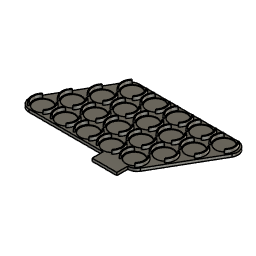
electrode_container_plate_rev_A_v1 (Autodesk Fusion 360 design; units mm, degrees)
Autodesk Fusion 360 part; units mm, degrees
note: some values were not read from the file. Chosen so that the rebuilt part matches the saved one: which bodies a step acts on. Set by a fixed rule: which sketch regions a step uses.
sketch "Sketch1" plane through (0, 0, 0) normal (0, 0, 1) x (1, 0, 0)
  circle A0 centre (0, 0) radius 8.55
  circle A1 centre (0, 0) radius 10
  line L0 (-7.0711, 7.0711) -> (7.0711, -7.0711)
  line L1 (-7.0711, -7.0711) -> (7.0711, 7.0711)
  line L2 (10, 0) -> (-10, 0) construction
  circle A2 centre (0, 0) radius 8
  dimension "d1" = 17.1
  dimension "d2" = 20
  dimension "d3" = 45
  dimension "d4" = 45
  dimension "d31" = 16
  constraint coincident A0.centre A1.centre
  constraint concentric A0 A1
  constraint coincident A1 L0.start
  constraint coincident A1 L0.end
  constraint coincident A1 L1.start
  constraint coincident A1 L1.end
  constraint midpoint A0.centre L1
  constraint midpoint A0.centre L0
  constraint coincident A1 L2.start
  constraint coincident A1 L2.end
  constraint horizontal L2
  measures "d1" diameter of A0
  measures "d2" diameter of A1
  measures "d3" angle of L1 L2
  measures "d4" angle of L0 L2
  measures "d31" diameter of A2
extrude "Extrude1" add sketch "Sketch1" along normal blind 3 draft -5 contours A0 A1 L0 L1 | A0 A1 L0 L1 picked at (9.4638, -0.8071) picked at (-7.307, -6.0626) makes body 1 at (9.2025, 3.6841, 1) makes body 2 at (-9.2025, 3.6841, 1)
pattern_linear "R-Pattern1" count 5 spacing 21 along (1, 0, 0) of bodies 2 1 makes body 3 at (30.2025, 3.6841, 1) makes body 4 at (51.2025, 3.6841, 1) makes body 5 at (72.2025, 3.6841, 1) makes body 6 at (93.2025, 3.6841, 1) makes body 7 at (11.7975, 3.6841, 1) makes body 8 at (32.7975, 3.6841, 1) makes body 9 at (53.7975, 3.6841, 1) makes body 10 at (74.7975, 3.6841, 1)
sketch "Sketch2" plane through (0, 0, 0) normal (0, 0, 1) x (1, 0, 0)
  line L0 (0, 0) -> (25.6285, 44.3898) construction
  line L1 (0, 0) -> (108.2634, 0) construction
  dimension "d11" = 60
  constraint coincident L0.start L1.start
  constraint horizontal L1
  measures "d11" angle of L0 L1
pattern_linear "R-Pattern2" count 4 spacing 20 along (0.5, 0.866025, 0) of bodies 6 1 3 5 10 2 7 9 8 4 makes body 11 at (19.2025, 21.0046, 1) makes body 12 at (29.2025, 38.3251, 1) makes body 13 at (39.2025, 55.6456, 1) makes body 14 at (0.7975, 21.0046, 1) makes body 15 at (10.7975, 38.3251, 1) makes body 16 at (20.7975, 55.6456, 1) makes body 17 at (40.2025, 21.0046, 1) makes body 18 at (50.2025, 38.3251, 1) makes body 19 at (60.2025, 55.6456, 1) makes body 20 at (61.2025, 21.0046, 1) makes body 21 at (71.2025, 38.3251, 1) makes body 22 at (81.2025, 55.6456, 1) makes body 23 at (82.2025, 21.0046, 1) makes body 24 at (92.2025, 38.3251, 1) makes body 25 at (102.2025, 55.6456, 1) makes body 26 at (103.2025, 21.0046, 1) makes body 27 at (113.2025, 38.3251, 1) makes body 28 at (123.2025, 55.6456, 1) makes body 29 at (21.7975, 21.0046, 1) makes body 30 at (31.7975, 38.3251, 1) makes body 31 at (41.7975, 55.6456, 1) makes body 32 at (42.7975, 21.0046, 1) makes body 33 at (52.7975, 38.3251, 1) makes body 34 at (62.7975, 55.6456, 1) makes body 35 at (63.7975, 21.0046, 1) makes body 36 at (73.7975, 38.3251, 1) makes body 37 at (83.7975, 55.6456, 1) makes body 38 at (84.7975, 21.0046, 1) makes body 39 at (94.7975, 38.3251, 1) makes body 40 at (104.7975, 55.6456, 1)
sketch "Sketch3" plane through (0, 0, 0) normal (0, 0, 1) x (1, 0, 0)
  line L0 (-18.2372, -9.0711) -> (22.2372, 61.0326)
  line L1 (22.2372, 61.0326) -> (132.2372, 61.0326)
  line L2 (132.2372, 61.0326) -> (91.7628, -9.0711)
  arc A0 (91.0686, -6.6974) -> (91.0686, 6.6974) centre (84, 0) ccw
  spline S0 degree 2 poles (91.0711, -7.0711) (91.0711, -6.883) (91.0686, -6.6974) knots 0.02979 0.02979 0.02979 0.332096 0.332096 0.332096
  arc A1 (91.0711, -7.0711) -> (91.0711, 7.0711) centre (84, 0) ccw
  spline S1 degree 2 poles (91.0711, 7.0711) (91.0711, 6.883) (91.0686, 6.6974) knots 0.02979 0.02979 0.02979 0.332096 0.332096 0.332096
  arc A2 (22.9314, 58.6589) -> (22.9314, 45.2641) centre (30, 51.9615) ccw
  spline S2 degree 2 poles (22.9289, 59.0326) (22.9289, 58.8445) (22.9314, 58.6589) knots 0.02979 0.02979 0.02979 0.332096 0.332096 0.332096
  arc A3 (22.9289, 59.0326) -> (22.9289, 44.8905) centre (30, 51.9615) ccw
  spline S3 degree 2 poles (22.9289, 44.8905) (22.9289, 45.0785) (22.9314, 45.2641) knots 0.02979 0.02979 0.02979 0.332096 0.332096 0.332096
  line L3 (94, 0) -> (97, 0) construction
  line L4 (20, 51.9615) -> (17, 51.9615) construction
  line L5 (-18.2372, -9.0711) -> (91.7628, -9.0711)
  point P0 (91.0711, -7.0711)
  point P1 (-7.0711, -7.0711)
  point P2 (22.9289, 59.0326)
  point P3 (20, 51.9615)
  point P4 (94, 0)
  dimension "d17" = 60
  dimension "d19" = 2
  dimension "d20" = 3
  dimension "d21" = 3
  dimension "d27" = 2
  dimension "d28" = 60
  constraint horizontal L1
  constraint midpoint A3 P3
  constraint midpoint A1 P4
  constraint coincident P4 L3.start
  constraint coincident L2 L3.end
  constraint horizontal L3
  constraint coincident P3 L4.start
  constraint coincident L0 L4.end
  constraint horizontal L4
  constraint horizontal L5
  constraint coincident L0.start L5.start
  measures "d17" angle of L1 L2
  measures "d19" distance of L1 P2
  measures "d20" distance of P3 L4.end
  measures "d21" distance of P4 L3.end
  measures "d27" distance of P1 L5
  measures "d28" angle of L0 L5
extrude "Extrude2" add sketch "Sketch3" against normal blind 2.5 contours L0 L1 L2 L5 | A0 S0 A1 S1 | A2 S2 A3 S3 bodies 1 2 3 4 5 6 7 8 9 10 11 12 13 14 15 16 17 18 19 20 21 22 23 24 25 26 27 28 29 30 31 32 33 34 35 36 37 38 39 40
sketch "Sketch4" plane through (0, 0, -2.5) normal (0, 0, -1) x (1, 0, 0)
  line L0 (91.7628, 9.0711) -> (-18.2372, 9.0711)
  line L1 (-18.2372, 9.0711) -> (22.2372, -61.0326)
  line L2 (22.2372, -61.0326) -> (132.2372, -61.0326)
  line L3 (132.2372, -61.0326) -> (91.7628, 9.0711)
  line L4 (96.9289, -41.7121) -> (97.9542, -40.6868)
  arc A0 (97.9542, -28.5953) -> (97.9542, -40.6868) centre (104, -34.641) ccw
  line L5 (97.9542, -28.5953) -> (96.9289, -27.5699)
  arc A1 (96.9289, -27.5699) -> (96.9289, -41.7121) centre (104, -34.641) ccw
  line L6 (85.9289, -59.0326) -> (86.9542, -58.0073)
  arc A2 (86.9542, -45.9158) -> (86.9542, -58.0073) centre (93, -51.9615) ccw
  line L7 (86.9542, -45.9158) -> (85.9289, -44.8905)
  arc A3 (85.9289, -44.8905) -> (85.9289, -59.0326) centre (93, -51.9615) ccw
  line L8 (65.9289, -24.3916) -> (66.9542, -23.3663)
  arc A4 (66.9542, -11.2747) -> (66.9542, -23.3663) centre (73, -17.3205) ccw
  line L9 (66.9542, -11.2747) -> (65.9289, -10.2494)
  arc A5 (65.9289, -10.2494) -> (65.9289, -24.3916) centre (73, -17.3205) ccw
  line L10 (54.9289, -41.7121) -> (55.9542, -40.6868)
  arc A6 (55.9542, -28.5953) -> (55.9542, -40.6868) centre (62, -34.641) ccw
  line L11 (55.9542, -28.5953) -> (54.9289, -27.5699)
  arc A7 (54.9289, -27.5699) -> (54.9289, -41.7121) centre (62, -34.641) ccw
  line L12 (43.9289, -59.0326) -> (44.9542, -58.0073)
  arc A8 (44.9542, -45.9158) -> (44.9542, -58.0073) centre (51, -51.9615) ccw
  line L13 (44.9542, -45.9158) -> (43.9289, -44.8905)
  arc A9 (43.9289, -44.8905) -> (43.9289, -59.0326) centre (51, -51.9615) ccw
  line L14 (23.9289, -24.3916) -> (24.9542, -23.3663)
  arc A10 (24.9542, -11.2747) -> (24.9542, -23.3663) centre (31, -17.3205) ccw
  line L15 (24.9542, -11.2747) -> (23.9289, -10.2494)
  arc A11 (23.9289, -10.2494) -> (23.9289, -24.3916) centre (31, -17.3205) ccw
  line L16 (111.0711, -27.5699) -> (110.0458, -28.5953)
  arc A12 (110.0458, -40.6868) -> (110.0458, -28.5953) centre (104, -34.641) ccw
  line L17 (110.0458, -40.6868) -> (111.0711, -41.7121)
  arc A13 (111.0711, -41.7121) -> (111.0711, -27.5699) centre (104, -34.641) ccw
  line L18 (100.0711, -44.8905) -> (99.0458, -45.9158)
  arc A14 (99.0458, -58.0073) -> (99.0458, -45.9158) centre (93, -51.9615) ccw
  line L19 (99.0458, -58.0073) -> (100.0711, -59.0326)
  arc A15 (100.0711, -59.0326) -> (100.0711, -44.8905) centre (93, -51.9615) ccw
  line L20 (80.0711, -10.2494) -> (79.0458, -11.2747)
  arc A16 (79.0458, -23.3663) -> (79.0458, -11.2747) centre (73, -17.3205) ccw
  line L21 (79.0458, -23.3663) -> (80.0711, -24.3916)
  arc A17 (80.0711, -24.3916) -> (80.0711, -10.2494) centre (73, -17.3205) ccw
  line L22 (69.0711, -27.5699) -> (68.0458, -28.5953)
  arc A18 (68.0458, -40.6868) -> (68.0458, -28.5953) centre (62, -34.641) ccw
  line L23 (68.0458, -40.6868) -> (69.0711, -41.7121)
  arc A19 (69.0711, -41.7121) -> (69.0711, -27.5699) centre (62, -34.641) ccw
  line L24 (58.0711, -44.8905) -> (57.0458, -45.9158)
  arc A20 (57.0458, -58.0073) -> (57.0458, -45.9158) centre (51, -51.9615) ccw
  line L25 (57.0458, -58.0073) -> (58.0711, -59.0326)
  arc A21 (58.0711, -59.0326) -> (58.0711, -44.8905) centre (51, -51.9615) ccw
  line L26 (38.0711, -10.2494) -> (37.0458, -11.2747)
  arc A22 (37.0458, -23.3663) -> (37.0458, -11.2747) centre (31, -17.3205) ccw
  line L27 (37.0458, -23.3663) -> (38.0711, -24.3916)
  arc A23 (38.0711, -24.3916) -> (38.0711, -10.2494) centre (31, -17.3205) ccw
  line L28 (12.9289, -41.7121) -> (13.9542, -40.6868)
  arc A24 (13.9542, -28.5953) -> (13.9542, -40.6868) centre (20, -34.641) ccw
  line L29 (13.9542, -28.5953) -> (12.9289, -27.5699)
  arc A25 (12.9289, -27.5699) -> (12.9289, -41.7121) centre (20, -34.641) ccw
  line L30 (37.0711, -44.8905) -> (36.0458, -45.9158)
  arc A26 (36.0458, -58.0073) -> (36.0458, -45.9158) centre (30, -51.9615) ccw
  line L31 (36.0458, -58.0073) -> (37.0711, -59.0326)
  arc A27 (37.0711, -59.0326) -> (37.0711, -44.8905) centre (30, -51.9615) ccw
  line L32 (17.0711, -10.2494) -> (16.0458, -11.2747)
  arc A28 (16.0458, -23.3663) -> (16.0458, -11.2747) centre (10, -17.3205) ccw
  line L33 (16.0458, -23.3663) -> (17.0711, -24.3916)
  arc A29 (17.0711, -24.3916) -> (17.0711, -10.2494) centre (10, -17.3205) ccw
  line L34 (55.9289, -7.0711) -> (56.9542, -6.0458)
  arc A30 (56.9542, 6.0458) -> (56.9542, -6.0458) centre (63, 0) ccw
  line L35 (56.9542, 6.0458) -> (55.9289, 7.0711)
  arc A31 (55.9289, 7.0711) -> (55.9289, -7.0711) centre (63, 0) ccw
  line L36 (13.9289, -7.0711) -> (14.9542, -6.0458)
  arc A32 (14.9542, 6.0458) -> (14.9542, -6.0458) centre (21, 0) ccw
  line L37 (14.9542, 6.0458) -> (13.9289, 7.0711)
  arc A33 (13.9289, 7.0711) -> (13.9289, -7.0711) centre (21, 0) ccw
  line L38 (70.0711, 7.0711) -> (69.0458, 6.0458)
  arc A34 (69.0458, -6.0458) -> (69.0458, 6.0458) centre (63, 0) ccw
  line L39 (69.0458, -6.0458) -> (70.0711, -7.0711)
  arc A35 (70.0711, -7.0711) -> (70.0711, 7.0711) centre (63, 0) ccw
  line L40 (28.0711, 7.0711) -> (27.0458, 6.0458)
  arc A36 (27.0458, -6.0458) -> (27.0458, 6.0458) centre (21, 0) ccw
  line L41 (27.0458, -6.0458) -> (28.0711, -7.0711)
  arc A37 (28.0711, -7.0711) -> (28.0711, 7.0711) centre (21, 0) ccw
  line L42 (7.0711, 7.0711) -> (6.0458, 6.0458)
  arc A38 (6.0458, -6.0458) -> (6.0458, 6.0458) centre (0, 0) ccw
  line L43 (6.0458, -6.0458) -> (7.0711, -7.0711)
  arc A39 (7.0711, -7.0711) -> (7.0711, 7.0711) centre (0, 0) ccw
  line L44 (-7.0711, -7.0711) -> (-6.0458, -6.0458)
  arc A40 (-6.0458, 6.0458) -> (-6.0458, -6.0458) centre (0, 0) ccw
  line L45 (-6.0458, 6.0458) -> (-7.0711, 7.0711)
  arc A41 (-7.0711, 7.0711) -> (-7.0711, -7.0711) centre (0, 0) ccw
  line L46 (49.0711, 7.0711) -> (48.0458, 6.0458)
  arc A42 (48.0458, -6.0458) -> (48.0458, 6.0458) centre (42, 0) ccw
  line L47 (48.0458, -6.0458) -> (49.0711, -7.0711)
  arc A43 (49.0711, -7.0711) -> (49.0711, 7.0711) centre (42, 0) ccw
  line L48 (91.0711, 7.0711) -> (90.0458, 6.0458)
  arc A44 (90.0458, -6.0458) -> (90.0458, 6.0458) centre (84, 0) ccw
  line L49 (90.0458, -6.0458) -> (91.0711, -7.0711)
  arc A45 (91.0711, -7.0711) -> (91.0711, 7.0711) centre (84, 0) ccw
  line L50 (34.9289, -7.0711) -> (35.9542, -6.0458)
  arc A46 (35.9542, 6.0458) -> (35.9542, -6.0458) centre (42, 0) ccw
  line L51 (35.9542, 6.0458) -> (34.9289, 7.0711)
  arc A47 (34.9289, 7.0711) -> (34.9289, -7.0711) centre (42, 0) ccw
  line L52 (76.9289, -7.0711) -> (77.9542, -6.0458)
  arc A48 (77.9542, 6.0458) -> (77.9542, -6.0458) centre (84, 0) ccw
  line L53 (77.9542, 6.0458) -> (76.9289, 7.0711)
  arc A49 (76.9289, 7.0711) -> (76.9289, -7.0711) centre (84, 0) ccw
  line L54 (27.0711, -27.5699) -> (26.0458, -28.5953)
  arc A50 (26.0458, -40.6868) -> (26.0458, -28.5953) centre (20, -34.641) ccw
  line L55 (26.0458, -40.6868) -> (27.0711, -41.7121)
  arc A51 (27.0711, -41.7121) -> (27.0711, -27.5699) centre (20, -34.641) ccw
  line L56 (2.9289, -24.3916) -> (3.9542, -23.3663)
  arc A52 (3.9542, -11.2747) -> (3.9542, -23.3663) centre (10, -17.3205) ccw
  line L57 (3.9542, -11.2747) -> (2.9289, -10.2494)
  arc A53 (2.9289, -10.2494) -> (2.9289, -24.3916) centre (10, -17.3205) ccw
  line L58 (22.9289, -59.0326) -> (23.9542, -58.0073)
  arc A54 (23.9542, -45.9158) -> (23.9542, -58.0073) centre (30, -51.9615) ccw
  line L59 (23.9542, -45.9158) -> (22.9289, -44.8905)
  arc A55 (22.9289, -44.8905) -> (22.9289, -59.0326) centre (30, -51.9615) ccw
  line L60 (48.0711, -27.5699) -> (47.0458, -28.5953)
  arc A56 (47.0458, -40.6868) -> (47.0458, -28.5953) centre (41, -34.641) ccw
  line L61 (47.0458, -40.6868) -> (48.0711, -41.7121)
  arc A57 (48.0711, -41.7121) -> (48.0711, -27.5699) centre (41, -34.641) ccw
  line L62 (59.0711, -10.2494) -> (58.0458, -11.2747)
  arc A58 (58.0458, -23.3663) -> (58.0458, -11.2747) centre (52, -17.3205) ccw
  line L63 (58.0458, -23.3663) -> (59.0711, -24.3916)
  arc A59 (59.0711, -24.3916) -> (59.0711, -10.2494) centre (52, -17.3205) ccw
  line L64 (79.0711, -44.8905) -> (78.0458, -45.9158)
  arc A60 (78.0458, -58.0073) -> (78.0458, -45.9158) centre (72, -51.9615) ccw
  line L65 (78.0458, -58.0073) -> (79.0711, -59.0326)
  arc A61 (79.0711, -59.0326) -> (79.0711, -44.8905) centre (72, -51.9615) ccw
  line L66 (90.0711, -27.5699) -> (89.0458, -28.5953)
  arc A62 (89.0458, -40.6868) -> (89.0458, -28.5953) centre (83, -34.641) ccw
  line L67 (89.0458, -40.6868) -> (90.0711, -41.7121)
  arc A63 (90.0711, -41.7121) -> (90.0711, -27.5699) centre (83, -34.641) ccw
  line L68 (101.0711, -10.2494) -> (100.0458, -11.2747)
  arc A64 (100.0458, -23.3663) -> (100.0458, -11.2747) centre (94, -17.3205) ccw
  line L69 (100.0458, -23.3663) -> (101.0711, -24.3916)
  arc A65 (101.0711, -24.3916) -> (101.0711, -10.2494) centre (94, -17.3205) ccw
  line L70 (121.0711, -44.8905) -> (120.0458, -45.9158)
  arc A66 (120.0458, -58.0073) -> (120.0458, -45.9158) centre (114, -51.9615) ccw
  line L71 (120.0458, -58.0073) -> (121.0711, -59.0326)
  arc A67 (121.0711, -59.0326) -> (121.0711, -44.8905) centre (114, -51.9615) ccw
  line L72 (33.9289, -41.7121) -> (34.9542, -40.6868)
  arc A68 (34.9542, -28.5953) -> (34.9542, -40.6868) centre (41, -34.641) ccw
  line L73 (34.9542, -28.5953) -> (33.9289, -27.5699)
  arc A69 (33.9289, -27.5699) -> (33.9289, -41.7121) centre (41, -34.641) ccw
  line L74 (44.9289, -24.3916) -> (45.9542, -23.3663)
  arc A70 (45.9542, -11.2747) -> (45.9542, -23.3663) centre (52, -17.3205) ccw
  line L75 (45.9542, -11.2747) -> (44.9289, -10.2494)
  arc A71 (44.9289, -10.2494) -> (44.9289, -24.3916) centre (52, -17.3205) ccw
  line L76 (64.9289, -59.0326) -> (65.9542, -58.0073)
  arc A72 (65.9542, -45.9158) -> (65.9542, -58.0073) centre (72, -51.9615) ccw
  line L77 (65.9542, -45.9158) -> (64.9289, -44.8905)
  arc A73 (64.9289, -44.8905) -> (64.9289, -59.0326) centre (72, -51.9615) ccw
  line L78 (75.9289, -41.7121) -> (76.9542, -40.6868)
  arc A74 (76.9542, -28.5953) -> (76.9542, -40.6868) centre (83, -34.641) ccw
  line L79 (76.9542, -28.5953) -> (75.9289, -27.5699)
  arc A75 (75.9289, -27.5699) -> (75.9289, -41.7121) centre (83, -34.641) ccw
  line L80 (86.9289, -24.3916) -> (87.9542, -23.3663)
  arc A76 (87.9542, -11.2747) -> (87.9542, -23.3663) centre (94, -17.3205) ccw
  line L81 (87.9542, -11.2747) -> (86.9289, -10.2494)
  arc A77 (86.9289, -10.2494) -> (86.9289, -24.3916) centre (94, -17.3205) ccw
  line L82 (106.9289, -59.0326) -> (107.9542, -58.0073)
  arc A78 (107.9542, -45.9158) -> (107.9542, -58.0073) centre (114, -51.9615) ccw
  line L83 (107.9542, -45.9158) -> (106.9289, -44.8905)
  arc A79 (106.9289, -44.8905) -> (106.9289, -59.0326) centre (114, -51.9615) ccw
  line L84 (-18.2372, 9.0711) -> (91.7628, 9.0711)
  line L85 (91.7628, 9.0711) -> (132.2372, -61.0326)
  line L86 (132.2372, -61.0326) -> (22.2372, -61.0326)
  line L87 (22.2372, -61.0326) -> (-18.2372, 9.0711)
extrude "Extrude3" cut sketch "Sketch4" against normal blind 1 contours L4 A0 L5 A1 | L6 A2 L7 A3 | L8 A4 L9 A5 | L10 A6 L11 A7 | L12 A8 L13 A9 | L14 A10 L15 A11 | L16 A12 L17 A13 | L18 A14 L19 A15 | L20 A16 L21 A17 | L22 A18 L23 A19 | L24 A20 L25 A21 | L26 A22 L27 A23 | L28 A24 L29 A25 | L30 A26 L31 A27 | L32 A28 L33 A29 | L34 A30 L35 A31 | L36 A32 L37 A33 | L38 A34 L39 A35 | L40 A36 L41 A37 | L42 A38 L43 A39 | L44 A40 L45 A41 | L46 A42 L47 A43 | L48 A44 L49 A45 | L50 A46 L51 A47 | L52 A48 L53 A49 | L54 A50 L55 A51 | L56 A52 L57 A53 | L58 A54 L59 A55 | L60 A56 L61 A57 | L62 A58 L63 A59 | L64 A60 L65 A61 | L66 A62 L67 A63 | L68 A64 L69 A65 | L70 A66 L71 A67 | L72 A68 L73 A69 | L74 A70 L75 A71 | L76 A72 L77 A73 | L78 A74 L79 A75 | L80 A76 L81 A77 | L82 A78 L83 A79 bodies 1
fillet "Fillet1" radius 8.5 4 edges at (-18.2372, -9.0711, -1.25) (91.7628, -9.0711, -1.25) (132.2372, 61.0326, -1.25) (22.2372, 61.0326, -1.25) on bodies 1
extrude "Extrude5" cut sketch "Sketch1" against normal blind 0.5 contours L0 L1 A2 | L0 L1 A2 | L0 L1 A2 | L0 L1 A2 bodies 1
pattern_linear "R-Pattern3" count 5 spacing 21 along (1, 0, 0) of "Extrude5"
pattern_linear "R-Pattern4" count 4 spacing 20 along (0.5, 0.866025, 0) of "Extrude5", "R-Pattern3"
sketch "Sketch5" plane through (0, 0, 0) normal (0, 0, 1) x (-1, 0, 0)
  circle A0 centre (-114, -51.9615) radius 8
  circle A1 centre (-93, -51.9615) radius 8
  circle A2 centre (-72, -51.9615) radius 8
  circle A3 centre (-51, -51.9615) radius 8
  circle A4 centre (-30, -51.9615) radius 8
  circle A5 centre (-104, -34.641) radius 8
  circle A6 centre (-83, -34.641) radius 8
  circle A7 centre (-62, -34.641) radius 8
  circle A8 centre (-41, -34.641) radius 8
  circle A9 centre (-20, -34.641) radius 8
  circle A10 centre (-94, -17.3205) radius 8
  circle A11 centre (-73, -17.3205) radius 8
  circle A12 centre (-52, -17.3205) radius 8
  circle A13 centre (-31, -17.3205) radius 8
  circle A14 centre (-10, -17.3205) radius 8
  circle A15 centre (-84, 0) radius 8
  circle A16 centre (-63, 0) radius 8
  circle A17 centre (-42, 0) radius 8
  circle A18 centre (-21, 0) radius 8
  circle A19 centre (0, 0) radius 8
  line L0 (-96.9289, -41.7121) -> (-97.9542, -40.6868)
  arc A20 (-97.9542, -40.6868) -> (-97.9542, -28.5953) centre (-104, -34.641) ccw
  line L1 (-97.9542, -28.5953) -> (-96.9289, -27.5699)
  arc A21 (-96.9289, -41.7121) -> (-96.9289, -27.5699) centre (-104, -34.641) ccw
  line L2 (-85.9289, -59.0326) -> (-86.9542, -58.0073)
  arc A22 (-86.9542, -58.0073) -> (-86.9542, -45.9158) centre (-93, -51.9615) ccw
  line L3 (-86.9542, -45.9158) -> (-85.9289, -44.8905)
  arc A23 (-85.9289, -59.0326) -> (-85.9289, -44.8905) centre (-93, -51.9615) ccw
  line L4 (-65.9289, -24.3916) -> (-66.9542, -23.3663)
  arc A24 (-66.9542, -23.3663) -> (-66.9542, -11.2747) centre (-73, -17.3205) ccw
  line L5 (-66.9542, -11.2747) -> (-65.9289, -10.2494)
  arc A25 (-65.9289, -24.3916) -> (-65.9289, -10.2494) centre (-73, -17.3205) ccw
  line L6 (-54.9289, -41.7121) -> (-55.9542, -40.6868)
  arc A26 (-55.9542, -40.6868) -> (-55.9542, -28.5953) centre (-62, -34.641) ccw
  line L7 (-55.9542, -28.5953) -> (-54.9289, -27.5699)
  arc A27 (-54.9289, -41.7121) -> (-54.9289, -27.5699) centre (-62, -34.641) ccw
  line L8 (-43.9289, -59.0326) -> (-44.9542, -58.0073)
  arc A28 (-44.9542, -58.0073) -> (-44.9542, -45.9158) centre (-51, -51.9615) ccw
  line L9 (-44.9542, -45.9158) -> (-43.9289, -44.8905)
  arc A29 (-43.9289, -59.0326) -> (-43.9289, -44.8905) centre (-51, -51.9615) ccw
  line L10 (-23.9289, -24.3916) -> (-24.9542, -23.3663)
  arc A30 (-24.9542, -23.3663) -> (-24.9542, -11.2747) centre (-31, -17.3205) ccw
  line L11 (-24.9542, -11.2747) -> (-23.9289, -10.2494)
  arc A31 (-23.9289, -24.3916) -> (-23.9289, -10.2494) centre (-31, -17.3205) ccw
  line L12 (-111.0711, -27.5699) -> (-110.0458, -28.5953)
  arc A32 (-110.0458, -28.5953) -> (-110.0458, -40.6868) centre (-104, -34.641) ccw
  line L13 (-110.0458, -40.6868) -> (-111.0711, -41.7121)
  arc A33 (-111.0711, -27.5699) -> (-111.0711, -41.7121) centre (-104, -34.641) ccw
  line L14 (-100.0711, -44.8905) -> (-99.0458, -45.9158)
  arc A34 (-99.0458, -45.9158) -> (-99.0458, -58.0073) centre (-93, -51.9615) ccw
  line L15 (-99.0458, -58.0073) -> (-100.0711, -59.0326)
  arc A35 (-100.0711, -44.8905) -> (-100.0711, -59.0326) centre (-93, -51.9615) ccw
  line L16 (-80.0711, -10.2494) -> (-79.0458, -11.2747)
  arc A36 (-79.0458, -11.2747) -> (-79.0458, -23.3663) centre (-73, -17.3205) ccw
  line L17 (-79.0458, -23.3663) -> (-80.0711, -24.3916)
  arc A37 (-80.0711, -10.2494) -> (-80.0711, -24.3916) centre (-73, -17.3205) ccw
  line L18 (-69.0711, -27.5699) -> (-68.0458, -28.5953)
  arc A38 (-68.0458, -28.5953) -> (-68.0458, -40.6868) centre (-62, -34.641) ccw
  line L19 (-68.0458, -40.6868) -> (-69.0711, -41.7121)
  arc A39 (-69.0711, -27.5699) -> (-69.0711, -41.7121) centre (-62, -34.641) ccw
  line L20 (-58.0711, -44.8905) -> (-57.0458, -45.9158)
  arc A40 (-57.0458, -45.9158) -> (-57.0458, -58.0073) centre (-51, -51.9615) ccw
  line L21 (-57.0458, -58.0073) -> (-58.0711, -59.0326)
  arc A41 (-58.0711, -44.8905) -> (-58.0711, -59.0326) centre (-51, -51.9615) ccw
  line L22 (-38.0711, -10.2494) -> (-37.0458, -11.2747)
  arc A42 (-37.0458, -11.2747) -> (-37.0458, -23.3663) centre (-31, -17.3205) ccw
  line L23 (-37.0458, -23.3663) -> (-38.0711, -24.3916)
  arc A43 (-38.0711, -10.2494) -> (-38.0711, -24.3916) centre (-31, -17.3205) ccw
  line L24 (-12.9289, -41.7121) -> (-13.9542, -40.6868)
  arc A44 (-13.9542, -40.6868) -> (-13.9542, -28.5953) centre (-20, -34.641) ccw
  line L25 (-13.9542, -28.5953) -> (-12.9289, -27.5699)
  arc A45 (-12.9289, -41.7121) -> (-12.9289, -27.5699) centre (-20, -34.641) ccw
  line L26 (-37.0711, -44.8905) -> (-36.0458, -45.9158)
  arc A46 (-36.0458, -45.9158) -> (-36.0458, -58.0073) centre (-30, -51.9615) ccw
  line L27 (-36.0458, -58.0073) -> (-37.0711, -59.0326)
  arc A47 (-37.0711, -44.8905) -> (-37.0711, -59.0326) centre (-30, -51.9615) ccw
  line L28 (-17.0711, -10.2494) -> (-16.0458, -11.2747)
  arc A48 (-16.0458, -11.2747) -> (-16.0458, -23.3663) centre (-10, -17.3205) ccw
  line L29 (-16.0458, -23.3663) -> (-17.0711, -24.3916)
  arc A49 (-17.0711, -10.2494) -> (-17.0711, -24.3916) centre (-10, -17.3205) ccw
  line L30 (-55.9289, -7.0711) -> (-56.9542, -6.0458)
  arc A50 (-56.9542, -6.0458) -> (-56.9542, 6.0458) centre (-63, 0) ccw
  line L31 (-56.9542, 6.0458) -> (-55.9289, 7.0711)
  arc A51 (-55.9289, -7.0711) -> (-55.9289, 7.0711) centre (-63, 0) ccw
  line L32 (-13.9289, -7.0711) -> (-14.9542, -6.0458)
  arc A52 (-14.9542, -6.0458) -> (-14.9542, 6.0458) centre (-21, 0) ccw
  line L33 (-14.9542, 6.0458) -> (-13.9289, 7.0711)
  arc A53 (-13.9289, -7.0711) -> (-13.9289, 7.0711) centre (-21, 0) ccw
  line L34 (-70.0711, 7.0711) -> (-69.0458, 6.0458)
  arc A54 (-69.0458, 6.0458) -> (-69.0458, -6.0458) centre (-63, 0) ccw
  line L35 (-69.0458, -6.0458) -> (-70.0711, -7.0711)
  arc A55 (-70.0711, 7.0711) -> (-70.0711, -7.0711) centre (-63, 0) ccw
  line L36 (-28.0711, 7.0711) -> (-27.0458, 6.0458)
  arc A56 (-27.0458, 6.0458) -> (-27.0458, -6.0458) centre (-21, 0) ccw
  line L37 (-27.0458, -6.0458) -> (-28.0711, -7.0711)
  arc A57 (-28.0711, 7.0711) -> (-28.0711, -7.0711) centre (-21, 0) ccw
  line L38 (-7.0711, 7.0711) -> (-6.0458, 6.0458)
  arc A58 (-6.0458, 6.0458) -> (-6.0458, -6.0458) centre (0, 0) ccw
  line L39 (-6.0458, -6.0458) -> (-7.0711, -7.0711)
  arc A59 (-7.0711, 7.0711) -> (-7.0711, -7.0711) centre (0, 0) ccw
  line L40 (7.0711, -7.0711) -> (6.0458, -6.0458)
  arc A60 (6.0458, -6.0458) -> (6.0458, 6.0458) centre (0, 0) ccw
  line L41 (6.0458, 6.0458) -> (7.0711, 7.0711)
  arc A61 (7.0711, -7.0711) -> (7.0711, 7.0711) centre (0, 0) ccw
  line L42 (-49.0711, 7.0711) -> (-48.0458, 6.0458)
  arc A62 (-48.0458, 6.0458) -> (-48.0458, -6.0458) centre (-42, 0) ccw
  line L43 (-48.0458, -6.0458) -> (-49.0711, -7.0711)
  arc A63 (-49.0711, 7.0711) -> (-49.0711, -7.0711) centre (-42, 0) ccw
  line L44 (-91.0711, 7.0711) -> (-90.0458, 6.0458)
  arc A64 (-90.0458, 6.0458) -> (-90.0458, -6.0458) centre (-84, 0) ccw
  line L45 (-90.0458, -6.0458) -> (-91.0711, -7.0711)
  arc A65 (-91.0711, 7.0711) -> (-91.0711, -7.0711) centre (-84, 0) ccw
  line L46 (-34.9289, -7.0711) -> (-35.9542, -6.0458)
  arc A66 (-35.9542, -6.0458) -> (-35.9542, 6.0458) centre (-42, 0) ccw
  line L47 (-35.9542, 6.0458) -> (-34.9289, 7.0711)
  arc A67 (-34.9289, -7.0711) -> (-34.9289, 7.0711) centre (-42, 0) ccw
  line L48 (-76.9289, -7.0711) -> (-77.9542, -6.0458)
  arc A68 (-77.9542, -6.0458) -> (-77.9542, 6.0458) centre (-84, 0) ccw
  line L49 (-77.9542, 6.0458) -> (-76.9289, 7.0711)
  arc A69 (-76.9289, -7.0711) -> (-76.9289, 7.0711) centre (-84, 0) ccw
  line L50 (-27.0711, -27.5699) -> (-26.0458, -28.5953)
  arc A70 (-26.0458, -28.5953) -> (-26.0458, -40.6868) centre (-20, -34.641) ccw
  line L51 (-26.0458, -40.6868) -> (-27.0711, -41.7121)
  arc A71 (-27.0711, -27.5699) -> (-27.0711, -41.7121) centre (-20, -34.641) ccw
  line L52 (-2.9289, -24.3916) -> (-3.9542, -23.3663)
  arc A72 (-3.9542, -23.3663) -> (-3.9542, -11.2747) centre (-10, -17.3205) ccw
  line L53 (-3.9542, -11.2747) -> (-2.9289, -10.2494)
  arc A73 (-2.9289, -24.3916) -> (-2.9289, -10.2494) centre (-10, -17.3205) ccw
  line L54 (-22.9289, -59.0326) -> (-23.9542, -58.0073)
  arc A74 (-23.9542, -58.0073) -> (-23.9542, -45.9158) centre (-30, -51.9615) ccw
  line L55 (-23.9542, -45.9158) -> (-22.9289, -44.8905)
  arc A75 (-22.9289, -59.0326) -> (-22.9289, -44.8905) centre (-30, -51.9615) ccw
  line L56 (-48.0711, -27.5699) -> (-47.0458, -28.5953)
  arc A76 (-47.0458, -28.5953) -> (-47.0458, -40.6868) centre (-41, -34.641) ccw
  line L57 (-47.0458, -40.6868) -> (-48.0711, -41.7121)
  arc A77 (-48.0711, -27.5699) -> (-48.0711, -41.7121) centre (-41, -34.641) ccw
  line L58 (-59.0711, -10.2494) -> (-58.0458, -11.2747)
  arc A78 (-58.0458, -11.2747) -> (-58.0458, -23.3663) centre (-52, -17.3205) ccw
  line L59 (-58.0458, -23.3663) -> (-59.0711, -24.3916)
  arc A79 (-59.0711, -10.2494) -> (-59.0711, -24.3916) centre (-52, -17.3205) ccw
  line L60 (-79.0711, -44.8905) -> (-78.0458, -45.9158)
  arc A80 (-78.0458, -45.9158) -> (-78.0458, -58.0073) centre (-72, -51.9615) ccw
  line L61 (-78.0458, -58.0073) -> (-79.0711, -59.0326)
  arc A81 (-79.0711, -44.8905) -> (-79.0711, -59.0326) centre (-72, -51.9615) ccw
  line L62 (-90.0711, -27.5699) -> (-89.0458, -28.5953)
  arc A82 (-89.0458, -28.5953) -> (-89.0458, -40.6868) centre (-83, -34.641) ccw
  line L63 (-89.0458, -40.6868) -> (-90.0711, -41.7121)
  arc A83 (-90.0711, -27.5699) -> (-90.0711, -41.7121) centre (-83, -34.641) ccw
  line L64 (-101.0711, -10.2494) -> (-100.0458, -11.2747)
  arc A84 (-100.0458, -11.2747) -> (-100.0458, -23.3663) centre (-94, -17.3205) ccw
  line L65 (-100.0458, -23.3663) -> (-101.0711, -24.3916)
  arc A85 (-101.0711, -10.2494) -> (-101.0711, -24.3916) centre (-94, -17.3205) ccw
  line L66 (-121.0711, -44.8905) -> (-120.0458, -45.9158)
  arc A86 (-120.0458, -45.9158) -> (-120.0458, -58.0073) centre (-114, -51.9615) ccw
  line L67 (-120.0458, -58.0073) -> (-121.0711, -59.0326)
  arc A87 (-121.0711, -44.8905) -> (-121.0711, -59.0326) centre (-114, -51.9615) ccw
  line L68 (-33.9289, -41.7121) -> (-34.9542, -40.6868)
  arc A88 (-34.9542, -40.6868) -> (-34.9542, -28.5953) centre (-41, -34.641) ccw
  line L69 (-34.9542, -28.5953) -> (-33.9289, -27.5699)
  arc A89 (-33.9289, -41.7121) -> (-33.9289, -27.5699) centre (-41, -34.641) ccw
  line L70 (-44.9289, -24.3916) -> (-45.9542, -23.3663)
  arc A90 (-45.9542, -23.3663) -> (-45.9542, -11.2747) centre (-52, -17.3205) ccw
  line L71 (-45.9542, -11.2747) -> (-44.9289, -10.2494)
  arc A91 (-44.9289, -24.3916) -> (-44.9289, -10.2494) centre (-52, -17.3205) ccw
  line L72 (-64.9289, -59.0326) -> (-65.9542, -58.0073)
  arc A92 (-65.9542, -58.0073) -> (-65.9542, -45.9158) centre (-72, -51.9615) ccw
  line L73 (-65.9542, -45.9158) -> (-64.9289, -44.8905)
  arc A93 (-64.9289, -59.0326) -> (-64.9289, -44.8905) centre (-72, -51.9615) ccw
  line L74 (-75.9289, -41.7121) -> (-76.9542, -40.6868)
  arc A94 (-76.9542, -40.6868) -> (-76.9542, -28.5953) centre (-83, -34.641) ccw
  line L75 (-76.9542, -28.5953) -> (-75.9289, -27.5699)
  arc A95 (-75.9289, -41.7121) -> (-75.9289, -27.5699) centre (-83, -34.641) ccw
  line L76 (-86.9289, -24.3916) -> (-87.9542, -23.3663)
  arc A96 (-87.9542, -23.3663) -> (-87.9542, -11.2747) centre (-94, -17.3205) ccw
  line L77 (-87.9542, -11.2747) -> (-86.9289, -10.2494)
  arc A97 (-86.9289, -24.3916) -> (-86.9289, -10.2494) centre (-94, -17.3205) ccw
  line L78 (-106.9289, -59.0326) -> (-107.9542, -58.0073)
  arc A98 (-107.9542, -58.0073) -> (-107.9542, -45.9158) centre (-114, -51.9615) ccw
  line L79 (-107.9542, -45.9158) -> (-106.9289, -44.8905)
  arc A99 (-106.9289, -59.0326) -> (-106.9289, -44.8905) centre (-114, -51.9615) ccw
  arc A100 (-27.1447, -61.0326) -> (-19.7834, -56.7826) centre (-27.1447, -52.5326) ccw
  line L80 (-19.7834, -56.7826) -> (10.876, -3.6789)
  arc A101 (10.876, -3.6789) -> (3.5148, 9.0711) centre (3.5148, 0.5711) ccw
  line L81 (3.5148, 9.0711) -> (-86.8553, 9.0711)
  arc A102 (-86.8553, 9.0711) -> (-94.2166, 4.8211) centre (-86.8553, 0.5711) ccw
  line L82 (-94.2166, 4.8211) -> (-124.876, -48.2826)
  arc A103 (-124.876, -48.2826) -> (-117.5148, -61.0326) centre (-117.5148, -52.5326) ccw
  line L83 (-117.5148, -61.0326) -> (-27.1447, -61.0326)
  line L84 (-41.6703, 9.0711) -> (-86.8553, 9.0711)
  line L85 (-86.8553, 9.0711) -> (-86.8553, 19.0711)
  line L86 (-86.8553, 19.0711) -> (3.5148, 19.0711)
  line L87 (3.5148, 19.0711) -> (3.5148, 9.0711)
  line L88 (-41.6703, 9.0711) -> (-41.6703, 19.0711)
  line L89 (3.5148, 9.0711) -> (-41.6703, 9.0711)
  line L90 (-19.0778, 9.0711) -> (-19.0778, 19.0711)
  line L91 (-64.2628, 9.0711) -> (-64.2628, 19.0711)
  dimension "d44" = 10
  constraint horizontal L84
  constraint vertical L85
  constraint horizontal L86
  constraint vertical L87
  constraint coincident A101.end L81.start
  constraint coincident L81.end A102.start
  constraint midpoint L86 L88.end
  constraint horizontal L89
  constraint midpoint L89 L90.start
  constraint coincident L86 L90.end
  constraint perpendicular L86 L90
  constraint midpoint L84 L91.start
  constraint coincident L86 L91.end
  constraint perpendicular L86 L91
  constraint vertical L88
  measures "d44" distance of A101.end L86.end
extrude "Extrude6" add sketch "Sketch5" against normal blind 2.5 contours L81 L84 L85 L86 L91 bodies 1
equation "d4 = d3"
equation "d17 = d28"
equation "d19 = d27"
equation "d21 = d20"
